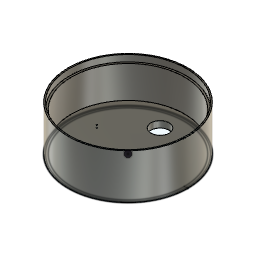
_bottom of mic base.243666c4-734c-4499-9f88-6792bb316d69 (Autodesk Fusion 360 design; units mm, degrees)
Autodesk Fusion 360 part; units mm, degrees
sketch "Sketch1" plane through (0, 0, 0) normal (0, 0, 1) x (1, 0, 0)
  circle A0 centre (0, 0) radius 45.5
  circle A1 centre (0, 0) radius 46.5
  circle A2 centre (0, 0) radius 44
  dimension "d1" = 91
  dimension "d2" = 93
  dimension "d3" = 88
  constraint coincident A0.centre A1.centre
  constraint concentric A1 A2
  measures "d1" diameter of A0
  measures "d2" diameter of A1
  measures "d3" diameter of A2
extrude "Extrude1" add sketch "Sketch1" along normal blind 5 contours A0 | A1 | A2
extrude "Extrude2" add sketch "Sketch1" along normal blind 30 contours A0
extrude "Extrude3" add sketch "Sketch1" along normal blind 35 contours A1
sketch "Sketch2" plane through (0, 0, 5) normal (0, 0, 1) x (-1, 0, 0)
  circle A0 centre (0, 0) radius 44
  line L0 (-24.5, 0) -> (24.5, 0) construction
  line L1 (24.5, 0) -> (24.5, 26) construction
  line L2 (24.5, 26) -> (-24.5, 26) construction
  line L3 (-24.5, 26) -> (-24.5, 0) construction
  circle A1 centre (-24.916, 26.2774) radius 0.5
  circle A2 centre (-25, 0) radius 0.5
  circle A3 centre (24.916, 26.2774) radius 0.5
  circle A4 centre (24.7236, -0.4472) radius 0.5
  dimension "d11" = 49
  dimension "d12" = 26
  dimension "d13" = 1
  dimension "d14" = 1
  dimension "d15" = 1
  dimension "d16" = 1
  constraint horizontal L0
  constraint vertical L1
  constraint horizontal L2
  constraint vertical L3
  constraint midpoint L0 A0.centre
  constraint coincident L2.end A1
  constraint coincident L0.start A2
  constraint coincident L1.end A3
  constraint coincident L0.end A4
  measures "d11" distance of L1.end L2.end
  measures "d12" distance of L0.start L2.end
  measures "d13" diameter of A1
  measures "d14" diameter of A2
  measures "d15" diameter of A3
  measures "d16" diameter of A4
extrude "Extrude4" add sketch "Sketch2" along normal blind 2 contours A1 | A2 | A3 | A4
sketch "Sketch3" plane through (0, 0, 5) normal (0, 0, 1) x (-1, 0, 0)
  circle A0 centre (-24.916, 26.2774) radius 0.5
  circle A1 centre (24.916, 26.2774) radius 0.5
  circle A2 centre (-25, 0) radius 0.5
  circle A3 centre (24.7236, -0.4472) radius 0.5
  circle A4 centre (0, 0) radius 44
  circle A5 centre (0, -25) radius 7.0711
extrude "Extrude5" cut sketch "Sketch3" against normal blind 6 contours A5
